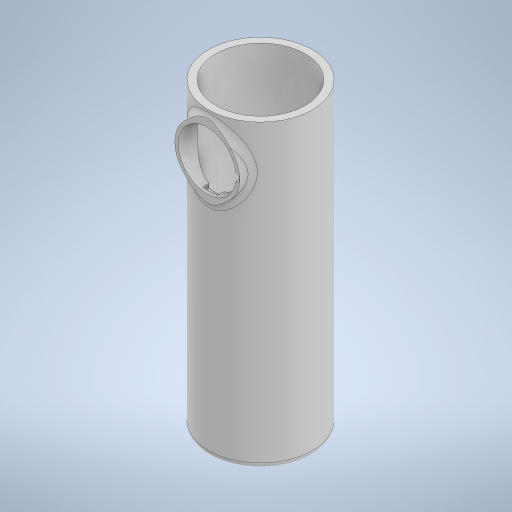
# Autodesk Inventor part: Flash_light
Saved by Autodesk Inventor 2024.2 (Build 282272000, 272)
## iProperties
Created: 2025-04-08
Part Number: Flash_light
Material: Generic
Document SubType Name: Modeling
Designer: Svend
Density: 1 g/cm^3
Appearance: Default
Author: Svend
Autodesk Inventor part; units mm, degrees
ref_plane "YZ Plane" through (0, 0, 0) normal (1, 0, 0) x (0, 1, 0)
ref_plane "XZ Plane" through (0, 0, 0) normal (0, 1, 0) x (-1, 0, 0)
sketch "Sketch1" plane through (0, 0, 0) normal (0, 1, 0) x (-1, 0, 0)
  circle A0 centre (0, 0) radius 15
  circle A1 centre (0, 0) radius 18
  dimension "d0" = 30
  dimension "d1" = 36
  constraints: 2 centre point, 2 coincident
  measures "d0" diameter of A0
  measures "d1" diameter of A1
extrude "Extrusion1" add sketch "Sketch1" along normal blind 4 contours A0 | A1
sketch "Sketch2" plane through (0, 4, 0) normal (0, -1, 0) x (1, 0, 0)
  circle A0 centre (0, 0) radius 18 projected
  circle A1 centre (0, 0) radius 15.5
  dimension "d17" = 2.5
  constraints: 1 centre point
  measures "d17" radial gap between concentric circles of A0 A1
extrude "Extrusion2" add sketch "Sketch2" against normal blind 100
ref_plane "Work Plane1" through (0, 0, 18.4) normal (0, 0, 1) x (1, 0, 0)
ref_plane "Work Plane2" through (0, 0, 18) normal (0, 0, 1) x (1, 0, 0)
sketch "Sketch3" plane through (0, 0, 18.4) normal (0, 0, 1) x (1, 0, 0)
  line L0 (16, 104) -> (-16, 104) construction
  line L1 (0, 104) -> (0, 89) construction
  circle A0 centre (0, 89) radius 10
  circle A1 centre (0, 89) radius 11.2
  line L2 (11, 90.2) -> (9.9277, 90.2)
  line L3 (9, 90.2) -> (9, 87.8) construction
  line L4 (9, 87.8) -> (9.9277, 87.8) construction
  line L5 (11, 87.8) -> (11, 90.2)
  line L6 (11, 90.2) -> (9, 87.8) construction
  line L7 (9, 90.2) -> (11, 87.8) construction
  line L8 (9.9277, 90.2) -> (9, 90.2) construction
  line L9 (9.9277, 87.8) -> (11, 87.8)
  point P0 (0, 0)
  point P1 (10, 89)
  dimension "d8" = 15
  dimension "d9" = 20
  dimension "d19" = 1.2
  dimension "d29" = 1
  dimension "d30" = 2.4
  constraints: 18 end point, 5 parallel, 3 midpoint, 3 point on circle, 2 centre point, 2 horizontal, 2 perpendicular, 1 coincident, 1 horizontal alignment, 1 vertical
  measures "d8" distance of L1.start L1.end
  measures "d9" diameter of A0
  measures "d19" radial gap between concentric circles of A1 A0
  measures "d29" distance from line of L5 A0.start
  measures "d30" distance of L5.start L2.start
extrude "Extrusion4" add sketch "Sketch3" against normal up to surface contours A0 | A0 L2 L5 L9 | A1 round surface about axis through (0, 0, 0) along (0, 1, 0) radius 18 far side no
extrude "Extrusion3" cut sketch "Sketch3" against normal blind 10 contours A0 | A0 L2 L5 L9
fillet "Fillet1" radius 3 3 edges at (8.5114, 81.7202, 15.8605) (8.5092, 96.2824, 15.8617) (-11.2, 88.9945, 14.0911)
fillet "Fillet2" radius 2 1 edges at (18, 0, 0)
ref_plane "Work Plane3" through (0, 0, 17.4) normal (0, 0, 1) x (1, 0, 0)
sketch "Sketch4" plane through (0, 0, 17.4) normal (0, 0, 1) x (1, 0, 0)
  line L0 (-4.6087, 102.1427) -> (-4.6087, 104) projected
  line L1 (-4.6087, 104) -> (4.6087, 104) projected
  line L2 (4.6087, 104) -> (4.6087, 102.1427) projected
  arc A0 (9.2736, 82.7198) -> (9.2736, 95.2802) centre (0, 89) ccw projected
  line L3 (4.6087, 75.8573) -> (4.6087, 2) projected
  line L4 (-4.6087, 2) -> (-4.6087, 75.8573) projected
  arc A1 (-9.2736, 95.2802) -> (-9.2736, 82.7198) centre (0, 89) ccw projected
  line L5 (0, 89) -> (-10, 89) construction
  line L6 (0, 89) -> (10, 89) construction
  line L7 (-2.5, 78) -> (2.5, 78)
  line L8 (2.5, 78) -> (2.5, 100)
  line L9 (2.5, 100) -> (-2.5, 100)
  line L10 (-2.5, 100) -> (-2.5, 78)
  line L11 (-2.5, 78) -> (2.5, 100) construction
  line L12 (2.5, 78) -> (-2.5, 100) construction
  line L13 (11, 90.2) -> (9.9277, 90.2) projected
  arc A2 (9.9277, 90.2) -> (9.9277, 87.8) centre (0, 89) ccw projected
  line L14 (9.9277, 87.8) -> (11, 87.8) projected
  line L15 (11, 87.8) -> (11, 90.2) projected
  point P0 (0, 0)
  dimension "d24" = 5
  dimension "d25" = 22
  constraints: 16 end point, 2 horizontal, 2 midpoint, 2 parallel, 1 horizontal alignment, 1 perpendicular, 1 point on line, 4 other
  measures "d24" distance of L9.end L8.end
  measures "d25" distance of L8.end L7.end
extrude "Extrusion5" cut sketch "Sketch4" against normal up to surface contours L10 A2 L8 L7 | L10 A2 L8 | L10 L9 L8 A2 round surface about axis through (0, 4, 0) along (0, 1, 0) radius 15.5 far side no
body "Solid1"
